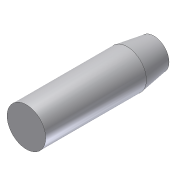
# Autodesk Inventor part: FE-00002-02
Saved by Autodesk Inventor 2012 (Build 160160000, 160)
## iProperties
Created: 2008-05-14
Part Number: FE-00002-02
Document SubType Name: Modeling
Designer: narosenberg
Density: 1 g/cm^3
Mass: 120.966 g
Surface Area: 152.426 cm^2
Volume: 120.966 cm^3
Material: Default
Author: narosenberg
Autodesk Inventor part; units mm, degrees
ref_plane "YZ Plane" through (0, 0, 0) normal (1, 0, 0) x (0, 1, 0)
ref_plane "XZ Plane" through (0, 0, 0) normal (0, 1, 0) x (-1, 0, 0)
ref_plane "XY Plane" through (0, 0, 0) normal (0, 0, 1) x (1, 0, 0)
sketch "Sketch1" plane through (0, 0, 0) normal (0, 0, 1) x (1, 0, 0)
  circle A0 centre (-4.8387, 12.596) radius 18.2563
  dimension "d0" = 36.5125
  constraints: 1 centre point
  measures "d0" diameter of A0
extrude "Extrusion1" add sketch "Sketch1" along normal blind 120.65
chamfer "Chamfer1" distance 3.9688 distance2 25.4 1 edges at (-23.095, 12.596, 0) measured on face at (1.1407, 16.9825, 0)
body "Solid1"
